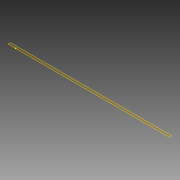
# Autodesk Inventor part: supporto_guide_lungo
Saved by Autodesk Inventor 2014 SP1 (Build 180222100, 222)
## iProperties
Created: 2015-04-08
Part Number: supporto_guide_lungo
Material: Generic
Document SubType Name: Modeling
Designer: Giorgio Nuzzo
Density: 1 g/cm^3
Appearance: Default
d0: 140,000 mm
d1: 45,000 mm
d5: 18,000 mm
d6: 25,000 mm
d7: 25,000 mm
d8: 4,000 mm
d9: 6,000 mm
d10: 45,000 mm
d11: 8,000 mm
d12: 8,000 mm
d14: 10,000 mm
d15: 0,00 deg
d16: 120,522 mm
Author: Giorgio Nuzzo
Autodesk Inventor part; units mm, degrees
ref_plane "YZ Plane" through (0, 0, 0) normal (1, 0, 0) x (0, 1, 0)
ref_plane "XZ Plane" through (0, 0, 0) normal (0, 1, 0) x (-1, 0, 0)
ref_plane "XY Plane" through (0, 0, 0) normal (0, 0, 1) x (1, 0, 0)
ref_plane "Work Plane1" through (0, 0, 0) normal (0, 0, 1) x (1, 0, 0)
sketch "Sketch1" plane through (0, 0, 0) normal (0, 0, 1) x (1, 0, 0)
  point P0 (0, 0)
ref_plane "Work Plane2" through (0, 0, 0) normal (0, 0, 1) x (1, 0, 0)
sketch "Sketch2" plane through (0, 0, 0) normal (0, 0, 1) x (1, 0, 0)
  line L0 (133.9999, 0) -> (0, 0) construction
  line L1 (133.9999, 0) -> (133.9999, 2) construction
  line L2 (0, 2) -> (133.9999, 2) construction
  line L3 (0, 0) -> (0, 2) construction
  line L4 (137.0698, 41) -> (137.0698, 2)
  line L5 (137.0698, 2) -> (-2.9302, 2)
  line L6 (-2.9302, 2) -> (-2.9302, 41)
  line L7 (-2.9302, 47) -> (137.0698, 2) construction
  line L8 (137.0698, 47) -> (-2.9302, 2) construction
  line L9 (22.0698, 29) -> (112.0698, 29)
  line L10 (22.0698, 29) -> (13.7788, 44.8537)
  line L11 (67.0698, 29) -> (67.0698, 47) construction
  line L12 (112.0698, 29) -> (120.3608, 44.8537)
  line L13 (3.0698, 47) -> (10.2342, 47)
  line L14 (123.9053, 47) -> (131.0698, 47)
  arc A0 (13.7788, 44.8537) -> (10.2342, 47) centre (10.2342, 43) ccw
  arc A1 (123.9053, 47) -> (120.3608, 44.8537) centre (123.9053, 43) ccw
  arc A2 (3.0698, 47) -> (-2.9302, 41) centre (3.0698, 41) ccw
  arc A3 (137.0698, 41) -> (131.0698, 47) centre (131.0698, 41) ccw
  circle A4 centre (6.8088, 39) radius 4
  circle A5 centre (127.3308, 39) radius 4
  point P0 (67.0698, 24.5)
  point P1 (12.6563, 47)
  point P2 (121.4832, 47)
  dimension "d0" = 140
  dimension "d1" = 45
  dimension "d6" = 25
  dimension "d7" = 25
  dimension "d8" = 4
  dimension "d9" = 6
  dimension "d10" = 45
  dimension "d11" = 8
  dimension "d12" = 8
  dimension "d16" = 120.522
  constraints: 22 end point, 8 point on circle, 8 point on line, 8 tangent, 6 centre point, 3 midpoint, 3 parallel, 2 equal radius, 2 horizontal, 2 perpendicular, 2 symmetric about line, 1 collinear, 1 other
  measures "d0" distance between parallel lines of L4 L6
  measures "d1" distance of L5.end L7.start
  measures "d6" distance from line of L6 L9.start
  measures "d7" distance from line of L4 L9.end
  measures "d8" radius of A0
  measures "d9" radius of A2
  measures "d10" distance between parallel lines of L5 L14
  measures "d11" diameter of A4
  measures "d12" distance from line of L13 A4.centre
  measures "d16" distance of A5.centre A4.centre
extrude "Extrusion1" add sketch "Sketch2" against normal blind 10
body "Solid1"
